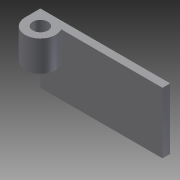
# Autodesk Inventor part: hingely
Saved by Autodesk Inventor 2011 (Build 150239000, 239)
## iProperties
Created: 2011-10-22
Part Number: hingely
Document SubType Name: Modeling
Designer: Matthew
Density: 1 g/cm^3
Author: Matthew
Autodesk Inventor part; units mm, degrees
ref_plane "YZ Plane" through (0, 0, 0) normal (1, 0, 0) x (0, 1, 0)
ref_plane "XZ Plane" through (0, 0, 0) normal (0, 1, 0) x (-1, 0, 0)
ref_plane "XY Plane" through (0, 0, 0) normal (0, 0, 1) x (1, 0, 0)
sketch "Sketch1" plane through (0, 0, 0) normal (0, 0, 1) x (1, 0, 0)
  line L0 (-11.9535, 4.9767) -> (38.8465, 4.9767)
  line L1 (38.8465, 4.9767) -> (38.8465, -20.4233)
  line L2 (38.8465, -20.4233) -> (-11.9535, -20.4233)
  line L3 (-11.9535, -20.4233) -> (-11.9535, 4.9767)
  point P0 (0, 0)
  dimension "d0" = 50.8
  dimension "d1" = 25.4
  constraints: 8 end point, 2 parallel, 1 horizontal, 1 perpendicular
  measures "d0" distance of L1.end L2.end
  measures "d1" distance of L0.end L1.end
extrude "Extrusion1" add sketch "Sketch1" along normal blind 3.175
sketch "Sketch2" plane through (-11.9535, 4.9767, 0) normal (0, 1, 0) x (1, 0, 0)
  line L0 (0, -3.175) -> (50.8, -3.175) projected
  line L1 (0, -3.175) -> (3.175, -3.175)
  line L2 (3.175, -3.175) -> (3.175, -6.35)
  circle A0 centre (3.175, -6.35) radius 3.175
  circle A1 centre (3.175, -6.35) radius 4.4901
  point P0 (11.9535, 0)
  dimension "d4" = 3.175
  dimension "d5" = 3.175
  constraints: 4 end point, 2 coincident, 1 perpendicular, 1 point on line, 1 vertical alignment, 5 other
  measures "d4" distance of L0.start L1.end
  measures "d5" distance of L1.end L2.end
extrude "Extrusion2" add sketch "Sketch2" against normal blind 12.7
sketch "Sketch3" plane through (-11.9535, 4.9767, 0) normal (0, 1, 0) x (1, 0, 0)
  line L0 (6.35, -3.175) -> (50.8, -3.175) projected
  arc A0 (0, -3.175) -> (6.35, -3.175) centre (3.175, -6.35) ccw projected
  line L1 (7.6651, -6.35) -> (7.6651, -3.175)
  point P0 (11.9535, 0)
  constraints: 2 end point, 1 perpendicular, 1 point on circle, 1 point on line, 1 tangent
extrude "Extrusion3" add sketch "Sketch3" against normal blind 12.7
sketch "Sketch4" plane through (-11.9535, 4.9767, 0) normal (0, 1, 0) x (1, 0, 0)
  line L0 (7.6651, -3.175) -> (50.8, -3.175) projected
  line L1 (50.8, 0) -> (50.8, -3.175) projected
  line L2 (0, 0) -> (50.8, 0) projected
  line L3 (0, 0) -> (0, -3.175) projected
  arc A0 (0, -3.175) -> (7.6651, -6.35) centre (3.175, -6.35) ccw projected
  line L4 (7.6651, -6.35) -> (7.6651, -3.175) projected
  line L5 (7.6651, -3.175) -> (7.6651, -12.2458)
  line L6 (3.175, -10.8401) -> (7.6651, -10.8401)
  point P0 (11.9535, 0)
  constraints: 4 end point, 1 collinear, 1 perpendicular, 1 point on circle, 1 point on line, 1 tangent
extrude "Extrusion4" add sketch "Sketch4" against normal blind 12.7 contours L5 L6 A0
sketch "Sketch5" plane through (-11.9535, 4.9767, 0) normal (0, 1, 0) x (1, 0, 0)
  arc A0 (0, -3.175) -> (3.175, -10.8401) centre (3.175, -6.35) ccw projected
  line L0 (3.175, -10.8401) -> (7.6651, -10.8401) projected
  line L1 (7.6651, -10.8401) -> (7.6651, -3.175) projected
  circle A1 centre (3.175, -6.35) radius 3.175 projected
  line L2 (7.6651, -3.175) -> (0, -3.175)
  point P0 (11.9535, 0)
  constraints: 2 end point
extrude "Extrusion5" cut sketch "Sketch5" against normal blind 25.4
sketch "Sketch6" plane through (-11.9535, 4.9767, 0) normal (0, 1, 0) x (1, 0, 0)
  line L0 (0, -3.175) -> (50.8, -3.175) projected
  line L1 (0, 0) -> (50.8, 0) projected
  line L2 (0, -3.175) -> (3.175, -3.175)
  line L3 (3.175, -3.175) -> (3.175, -6.35)
  circle A0 centre (3.175, -6.35) radius 3.175
  circle A1 centre (3.175, -6.35) radius 6.35
  point P0 (11.9535, 0)
  dimension "d14" = 3.175
  dimension "d15" = 3.175
  constraints: 4 end point, 2 coincident, 1 centre point, 1 perpendicular, 1 point on line, 1 tangent, 1 vertical alignment, 2 other
  measures "d14" distance of L0.start L2.end
  measures "d15" distance of L2.end L3.end
extrude "Extrusion6" add sketch "Sketch6" against normal blind 12.7
sketch "Sketch7" plane through (-11.9535, 4.9767, 0) normal (0, 1, 0) x (1, 0, 0)
  line L0 (0, 0) -> (0, -0.8507) projected
  arc A0 (0, -0.8507) -> (8.6743, -3.175) centre (3.175, -6.35) ccw projected
  line L1 (-3.175, -6.35) -> (-3.175, 0)
  line L2 (0, 0) -> (-3.175, 0)
  point P0 (11.9535, 0)
  constraints: 4 end point, 1 parallel, 1 perpendicular, 1 point on circle, 1 tangent
extrude "Extrusion7" add sketch "Sketch7" against normal blind 12.7
body "Solid1"
